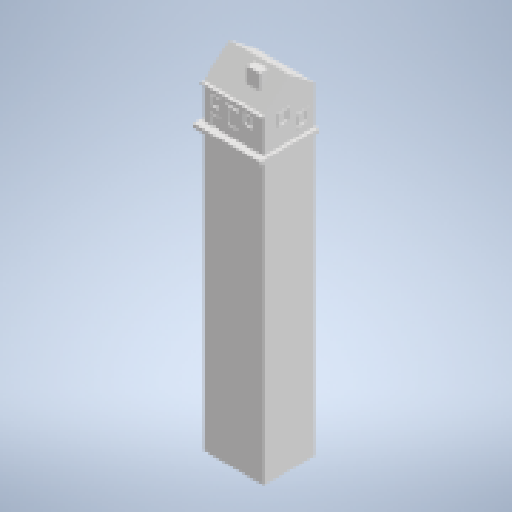
# Autodesk Inventor part: 屋1 物3
Saved by Autodesk Inventor 2024 (Build 280153000, 153)
## iProperties
Created: 2024-05-23
Part Number: 屋1 物3
Material: 一般
Document SubType Name: Modeling
Designer: User
Density: 1 g/cm^3
Appearance: 預設
Author: User
Autodesk Inventor part; units mm, degrees
ref_plane "YZ Plane" through (0, 0, 0) normal (1, 0, 0) x (0, 1, 0)
ref_plane "XZ Plane" through (0, 0, 0) normal (0, 1, 0) x (-1, 0, 0)
sketch "草圖1" plane through (0, 0, 0) normal (1, 0, 0) x (0, 1, 0)
  line L0 (0, 0) -> (-6.4572, 7.1039)
  line L1 (-6.4572, 7.1039) -> (-6.4572, 8.1039)
  line L2 (-6.4572, 8.1039) -> (-6.9572, 8.1039)
  line L3 (-6.9572, 8.1039) -> (-6.9572, 7.1039)
  line L4 (-6.9572, 7.1039) -> (-16.5572, 7.1039)
  line L5 (-16.5572, 7.1039) -> (-16.5572, 9.1039)
  line L6 (-16.5572, 9.1039) -> (-17.5572, 9.1039)
  line L7 (-17.5572, 9.1039) -> (-17.5572, 0)
  line L8 (0, 0) -> (-5.811, -7.5155)
  line L9 (-5.811, -7.5155) -> (-17.5572, -7.5155)
  line L10 (-17.5572, -7.5155) -> (-17.5572, 0)
  dimension "d0" = 9.6
  dimension "d1" = 1
  dimension "d2" = 0.5
  dimension "d3" = 9.6
  dimension "d4" = 2
  dimension "d5" = 1
  dimension "d6" = 9.5
  constraints: 22 end point, 6 perpendicular, 2 horizontal, 1 vertical
  measures "d0" distance of L0.start L0.end
  measures "d1" distance of L0.end L1.end
  measures "d2" distance of L1.end L2.end
  measures "d3" distance of L3.end L4.end
  measures "d4" distance of L4.end L5.end
  measures "d5" distance of L5.end L6.end
  measures "d6" distance of L0.start L8.end
extrude "擠出1" add sketch "草圖1" along normal blind 17
sketch "草圖2" plane through (0, 0, 0) normal (-1, 0, 0) x (0, 0, 1)
  line L0 (1.3244, -10.5521) -> (3.3244, -10.5521)
  line L1 (3.3244, -10.5521) -> (3.3244, -8.5521)
  line L2 (3.3244, -8.5521) -> (1.3244, -8.5521)
  line L3 (1.3244, -8.5521) -> (1.3244, -10.5521)
  line L4 (1.3244, -10.5521) -> (3.3244, -8.5521) construction
  line L5 (3.3244, -10.5521) -> (1.3244, -8.5521) construction
  line L6 (0.8244, -8.5521) -> (3.8244, -8.5521)
  line L7 (3.8244, -8.5521) -> (3.8244, -7.9272)
  line L8 (3.8244, -7.9272) -> (0.8244, -7.9272)
  line L9 (0.8244, -7.9272) -> (0.8244, -8.5521)
  line L10 (1.2244, -10.6521) -> (3.4244, -10.6521)
  line L11 (3.4244, -10.6521) -> (3.4244, -8.4521)
  line L12 (3.4244, -8.4521) -> (1.2244, -8.4521)
  line L13 (1.2244, -8.4521) -> (1.2244, -10.6521)
  line L14 (1.2244, -10.6521) -> (3.4244, -8.4521) construction
  line L15 (3.4244, -10.6521) -> (1.2244, -8.4521) construction
  point P0 (0, 0)
  point P1 (2.3244, -9.5521)
  point P2 (0.8244, -8.2396)
  point P3 (1.2244, -8.5521)
  point P4 (3.4244, -8.5521)
  dimension "d9" = 0.5
  dimension "d10" = 0.5
  dimension "d15" = 0.1
  dimension "d16" = 0.1
  dimension "d17" = 0.1
  dimension "d18" = 0.1
  dimension "d19" = 2
  constraints: 32 end point, 6 parallel, 5 midpoint, 3 horizontal, 3 perpendicular, 1 point on line
  measures "d9" distance between parallel lines of L1 L7
  measures "d10" distance from line of point (0.824, -8.24) L3
  measures "d15" distance between parallel lines of L1 L11
  measures "d16" distance between parallel lines of L13 L3
  measures "d17" distance between parallel lines of L6 L12
  measures "d18" distance between parallel lines of L2 L12
  measures "d19" distance between parallel lines of L2 L0
extrude "擠出2" add sketch "草圖2" along normal blind 0.5 contours L6 L13 L12 L11 L2 | L6 L9 L8 L7 L11 L12 L13
extrude "擠出3" cut sketch "草圖2" against normal blind 0.5 contours L3 L2 L1 L0
extrude "擠出4" add sketch "草圖2" along normal blind 0.3 contours L0 L1 L6 L11 L10 L13 L3
sketch "草圖3" plane through (0, -16.5572, 7.1039) normal (0, 0, 1) x (1, 0, 0)
  line L0 (2.4891, 7.7612) -> (4.5073, 7.7612)
  line L1 (4.5073, 7.7612) -> (4.5073, 5.2048)
  line L2 (4.5073, 5.2048) -> (2.4891, 5.2048)
  line L3 (2.4891, 5.2048) -> (2.4891, 7.7612)
  line L4 (0, 0) -> (17, 0) projected
  line L5 (2.4891, 0) -> (4.5073, 0)
  line L6 (4.5073, 0) -> (4.5073, 3.1193)
  line L7 (4.5073, 3.1193) -> (2.4891, 3.1193)
  line L8 (2.4891, 3.1193) -> (2.4891, 0)
  line L9 (6.761, 6.8866) -> (9.6873, 6.8866)
  line L10 (9.6873, 6.8866) -> (9.6873, 2.6148)
  line L11 (9.6873, 2.6148) -> (6.761, 2.6148)
  line L12 (6.761, 2.6148) -> (6.761, 6.8866)
  line L13 (11.6046, 7.7612) -> (13.8583, 7.7612)
  line L14 (13.8583, 7.7612) -> (13.8583, 5.2048)
  line L15 (13.8583, 5.2048) -> (11.6046, 5.2048)
  line L16 (11.6046, 5.2048) -> (11.6046, 7.7612)
  point P0 (0, 16.5572)
  constraints: 32 end point, 8 parallel, 5 point on line, 4 horizontal, 4 perpendicular
extrude "擠出5" cut sketch "草圖3" against normal blind 0.3
sketch "草圖4" plane through (0, -16.5572, 7.1039) normal (0, 0, 1) x (1, 0, 0)
  line L0 (0, 0) -> (17, 0) projected
  line L1 (2.2891, 0) -> (4.7073, 0)
  line L2 (4.7073, 0) -> (4.7073, 3.3193)
  line L3 (4.7073, 3.3193) -> (2.2891, 3.3193)
  line L4 (2.2891, 3.3193) -> (2.2891, 0)
  line L5 (6.561, 6.8866) -> (9.8873, 6.8866)
  line L6 (9.8873, 6.8866) -> (9.8873, 7.667)
  line L7 (9.8873, 7.667) -> (6.561, 7.667)
  line L8 (6.561, 7.667) -> (6.561, 6.8866)
  line L9 (6.761, 2.6148) -> (6.761, 6.8866) projected
  line L10 (9.6873, 6.8866) -> (9.6873, 2.6148) projected
  line L11 (4.5073, 3.1193) -> (4.5073, 0) projected
  line L12 (2.4891, 0) -> (2.4891, 3.1193) projected
  line L13 (2.4891, 3.1193) -> (4.5073, 3.1193) projected
  line L14 (2.2891, 7.9612) -> (4.7073, 7.9612)
  line L15 (4.7073, 7.9612) -> (4.7073, 5.0048)
  line L16 (4.7073, 5.0048) -> (2.2891, 5.0048)
  line L17 (2.2891, 5.0048) -> (2.2891, 7.9612)
  line L18 (11.4046, 7.9612) -> (14.0583, 7.9612)
  line L19 (14.0583, 7.9612) -> (14.0583, 5.0048)
  line L20 (14.0583, 5.0048) -> (11.4046, 5.0048)
  line L21 (11.4046, 5.0048) -> (11.4046, 7.9612)
  line L22 (11.6046, 7.7612) -> (13.8583, 7.7612) projected
  line L23 (13.8583, 7.7612) -> (13.8583, 5.2048) projected
  line L24 (11.6046, 5.2048) -> (11.6046, 7.7612) projected
  line L25 (13.8583, 5.2048) -> (11.6046, 5.2048) projected
  line L26 (4.5073, 7.7612) -> (4.5073, 5.2048) projected
  line L27 (4.5073, 5.2048) -> (2.4891, 5.2048) projected
  line L28 (2.4891, 5.2048) -> (2.4891, 7.7612) projected
  line L29 (2.4891, 7.7612) -> (4.5073, 7.7612)
  line L30 (4.5073, 7.7612) -> (4.5073, 5.2048)
  line L31 (4.5073, 5.2048) -> (2.4891, 5.2048)
  line L32 (2.4891, 5.2048) -> (2.4891, 7.7612)
  line L33 (2.4891, 3.1193) -> (4.5073, 3.1193)
  line L34 (4.5073, 3.1193) -> (4.5073, 0)
  line L35 (4.5073, 0) -> (2.4891, 0)
  line L36 (2.4891, 0) -> (2.4891, 3.1193)
  line L37 (11.6046, 7.7612) -> (13.8583, 7.7612)
  line L38 (13.8583, 7.7612) -> (13.8583, 5.2048)
  line L39 (13.8583, 5.2048) -> (11.6046, 5.2048)
  line L40 (11.6046, 5.2048) -> (11.6046, 7.7612)
  point P0 (0, 16.5572)
  dimension "d24" = 0.2
  dimension "d25" = 0.2
  dimension "d26" = 0.2
  dimension "d27" = 0.2
  dimension "d28" = 0.2
  dimension "d29" = 0.2
  dimension "d30" = 0.2
  dimension "d31" = 0.2
  dimension "d32" = 0.2
  dimension "d33" = 0.2
  dimension "d34" = 0.2
  dimension "d35" = 0.2
  constraints: 56 end point, 14 parallel, 7 horizontal, 7 perpendicular, 3 point on line
  measures "d24" distance between parallel lines of L9 L8
  measures "d25" distance between parallel lines of L10 L6
  measures "d26" distance between parallel lines of L11 L2
  measures "d27" distance between parallel lines of L12 L4
  measures "d28" distance between parallel lines of L13 L3
  measures "d29" distance between parallel lines of L22 L18
  measures "d30" distance between parallel lines of L23 L19
  measures "d31" distance between parallel lines of L21 L24
  measures "d32" distance between parallel lines of L25 L20
  measures "d33" distance between parallel lines of L15 L26
  measures "d34" distance between parallel lines of L16 L27
  measures "d35" distance between parallel lines of L28 L17
extrude "擠出6" add sketch "草圖4" along normal blind 0.2 contours L4 L3 L2 L0 L11 L13 L12 | L14 L15 L16 L17 | L18 L19 L20 L21
extrude "擠出7" add sketch "草圖4" along normal blind 0.5 contours L8 L7 L6 L5
sketch "草圖5" plane through (17, 0, 0) normal (1, 0, 0) x (0, 0, -1)
  line L0 (-2.8354, -8.2564) -> (-0.2487, -8.2564)
  line L1 (-0.2487, -8.2564) -> (-0.2487, -11.3114)
  line L2 (-0.2487, -11.3114) -> (-2.8354, -11.3114)
  line L3 (-2.8354, -11.3114) -> (-2.8354, -8.2564)
  line L4 (2.2042, -10.9992) -> (5.1699, -10.9992)
  line L5 (5.1699, -10.9992) -> (5.1699, -14.1433)
  line L6 (5.1699, -14.1433) -> (2.2042, -14.1433)
  line L7 (2.2042, -14.1433) -> (2.2042, -10.9992)
  line L8 (-3.0354, -8.0564) -> (-0.0487, -8.0564)
  line L9 (-0.0487, -8.0564) -> (-0.0487, -11.5114)
  line L10 (-0.0487, -11.5114) -> (-3.0354, -11.5114)
  line L11 (-3.0354, -11.5114) -> (-3.0354, -8.0564)
  line L12 (2.0042, -10.7992) -> (5.3699, -10.7992)
  line L13 (5.3699, -10.7992) -> (5.3699, -14.3433)
  line L14 (5.3699, -14.3433) -> (2.0042, -14.3433)
  line L15 (2.0042, -14.3433) -> (2.0042, -10.7992)
  point P0 (0, 0)
  dimension "d40" = 0.2
  dimension "d41" = 0.2
  dimension "d42" = 0.2
  dimension "d43" = 0.2
  dimension "d44" = 0.2
  dimension "d45" = 0.2
  dimension "d46" = 0.2
  dimension "d47" = 0.2
  constraints: 32 end point, 8 horizontal, 8 parallel, 4 perpendicular, 4 vertical, 8 other
  measures "d40" distance between parallel lines of L0 L8
  measures "d41" distance between parallel lines of L11 L3
  measures "d42" distance between parallel lines of L9 L1
  measures "d43" distance between parallel lines of L10 L2
  measures "d44" distance between parallel lines of L4 L12
  measures "d45" distance between parallel lines of L13 L5
  measures "d46" distance between parallel lines of L14 L6
  measures "d47" distance between parallel lines of L15 L7
extrude "擠出8" cut sketch "草圖5" against normal blind 0.3 contours L0 L1 L2 L3 | L4 L5 L6 L7
extrude "擠出9" add sketch "草圖5" along normal blind 0.2
sketch "草圖6" plane through (0, -17.5572, -7.5155) normal (0, -1, 0) x (1, 0, 0)
  line L0 (0, 0) -> (0, 7.5155) projected
  line L1 (17, 7.5155) -> (17, 14.6194) projected
  line L2 (0, 0) -> (17, 0)
  line L3 (17, 0) -> (17, 14.6194)
  line L4 (17, 14.6194) -> (0, 14.6194)
  line L5 (0, 14.6194) -> (0, 0)
  constraints: 8 end point, 2 parallel, 1 horizontal, 1 perpendicular
extrude "擠出10" add sketch "草圖6" along normal blind 78
sketch "草圖7" plane through (0, 0, 0) normal (-1, 0, 0) x (0, 0, 1)
  line L0 (9.1039, -16.5572) -> (9.1039, -17.5572) projected
  line L1 (-7.5155, -5.811) -> (-7.5155, -95.5572) projected
  line L2 (9.1039, -17.5572) -> (-7.5155, -17.5572)
  line L3 (-7.5155, -17.5572) -> (-7.5155, -16.5572)
  line L4 (-7.5155, -16.5572) -> (9.1039, -16.5572)
  line L5 (9.1039, -16.5572) -> (9.1039, -17.5572)
  point P0 (0, 0)
  point P1 (-7.5155, -17.5572)
  dimension "d54" = 1
  constraints: 8 end point, 2 parallel, 1 horizontal, 1 perpendicular, 1 point on line
  measures "d54" distance of L2.end L3.end
extrude "擠出11" add sketch "草圖7" along normal blind 1
ref_plane "工作平面1" through (8.5, 0, 0) normal (-1, 0, 0) x (0, 0, 1)
mirror "鏡射1" about plane through (8.5, 0, 0) normal (-1, 0, 0) of "擠出11"
sketch "草圖8" plane through (0, -17.5572, 7.1039) normal (0, -1, 0) x (1, 0, 0)
  line L0 (9.431, -2.7696) -> (13.1296, -2.7696)
  line L1 (13.1296, -2.7696) -> (13.1296, -5.0596)
  line L2 (13.1296, -5.0596) -> (9.431, -5.0596)
  line L3 (9.431, -5.0596) -> (9.431, -2.7696)
  point P0 (0, -7.1039)
  constraints: 8 end point, 2 parallel, 1 horizontal, 1 perpendicular
extrude "擠出12" add sketch "草圖8" against normal blind 18
